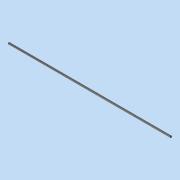
# Autodesk Inventor part: midshipsThreadedRodThread_5_40
Saved by Autodesk Inventor 2017 (Build 210142000, 142)
## iProperties
Created: 2016-10-29
Part Number: midshipsThreadedRodThread_5_40
Material: Stainless Steel, Polished
Document SubType Name: Modeling
Designer: techn
Density: 8 g/cm^3
Appearance: Stainless - Polished
Author: techn
Autodesk Inventor part; units mm, degrees
ref_plane "YZ Plane" through (0, 0, 0) normal (1, 0, 0) x (0, 1, 0)
ref_plane "XZ Plane" through (0, 0, 0) normal (0, 1, 0) x (-1, 0, 0)
ref_plane "XY Plane" through (0, 0, 0) normal (0, 0, 1) x (1, 0, 0)
sketch "Sketch1" plane through (0, 0, 0) normal (1, 0, 0) x (0, 1, 0)
  circle A0 centre (0, 0) radius 1.5875
  dimension "d0" = 3.175
  constraints: 1 centre point, 1 coincident
  measures "d0" diameter of A0
extrude "Extrusion1" add sketch "Sketch1" along normal blind 294.64
thread "Thread1" size "5-40 UNC" class "2A" standard "ANSI Unified Screw Threads" full length
body "Solid1"
